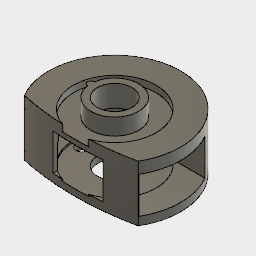
support rotacteur (Autodesk Fusion 360 design; units mm, degrees)
Autodesk Fusion 360 part; units mm, degrees
sketch "Sketch1" plane through (0, 0, 0) normal (0, 1, 0) x (1, 0, 0)
  circle A0 centre (0, 0) radius 7.25
  dimension "d1" = 14.5
  measures "d1" diameter of A0
extrude "Extrude1" add sketch "Sketch1" along normal blind 5 makes body 1
sketch "Sketch2" plane through (0, 0, 0) normal (0, 1, 0) x (1, 0, 0)
  circle A0 centre (0, 0) radius 20
  circle A1 centre (0, 0) radius 12.5
  dimension "d4" = 40
  dimension "d5" = 25
  measures "d4" diameter of A0
  measures "d5" diameter of A1
extrude "Extrude2" add sketch "Sketch2" against normal blind 15 separate body makes body 2
move_face "OffsetFaces1" offset 2 1 faces at (17.379, 0, 1.6146) on bodies 2
sketch "Sketch3" plane through (0, 5, 0) normal (0, 1, 0) x (-1, 0, 0)
  circle A0 centre (0, 0) radius 7.25
  circle A1 centre (0, 0) radius 5.25
  dimension "d9" = 10.5
  measures "d9" diameter of A1
extrude "Extrude3" cut sketch "Sketch3" against normal blind 20 contours A1 bodies 1
extrude "Extrude4" add sketch "Sketch2" against normal blind 2 contours A1 bodies 1 2
extrude "Extrude5" cut sketch "Sketch3" against normal blind 25 contours A1 bodies 1
extrude "Extrude6" add 1 faces at (10.0172, -2, 0.8818) along direction (0, -1, 0) blind 13 on bodies 1 bodies 1
cylinder "CylinderPrimitive1" add diameter 25 height 10 placed x (1, 0, 0) y (0, 0, 1) z (0, -1, 0) at (0, -15, 0) separate body makes body 3
move_body "MoveBody1" bodies 3 to x (1, 0, 0) y (0, 1, 0) z (0, 0, 1) at (0, 10, 0)
move_face "OffsetFaces2" offset -2 1 faces at (-3.3879, -15, -0.621) on bodies 3
combine "Combine1" operation cut target body 1 tool bodies 3
ref_plane "WorkPlane1" through (0, -6.5, 0) normal (0, -1, 0) x (-1, 0, 0)
sketch "Sketch5" plane through (0, -6.5, 0) normal (0, -1, 0) x (1, 0, 0)
  line L0 (-23, -8) -> (-65, -8)
  line L1 (-65, -8) -> (-65, 7)
  line L2 (-65, 7) -> (-23, 7)
  line L3 (-23, 7) -> (-23, -8)
  line L4 (-7, -22.2294) -> (8, -22.2294)
  line L5 (8, -22.2294) -> (8, -68)
  line L6 (8, -68) -> (-7, -68)
  line L7 (-7, -68) -> (-7, -22.2294)
  dimension "d21" = 15
  measures "d21" distance of L0.start L2.end
extrude "Extrude7" add sketch "Sketch5" along normal blind 6 separate body contours L0 L1 L2 L3 makes body 4
move_face "OffsetFaces3" offset 5 1 faces at (-51, -6.5, -3) on bodies 4
move_face "OffsetFaces4" offset 3 1 faces at (-51, -5.1667, 7) on bodies 4
move_face "OffsetFaces5" offset 2 1 faces at (-37, -5.1667, -8) on bodies 4
move_body "MoveBody2" bodies 4 to x (1, 0, 0) y (0, 1, 0) z (0, 0, 1) at (44, 0, 0)
extrude "Extrude8" add sketch "Sketch5" along normal blind 6 separate body contours L4 L5 L6 L7 makes body 5
extrude "Extrude9" add sketch "Sketch5" against normal blind 5 contours L4 L5 L6 L7 bodies 5
move_body "MoveBody3" bodies 5 to x (1, 0, 0) y (0, 1, 0) z (0, 0, 1) at (0, 0, 47)
combine "Combine2" operation cut target body 1 tool bodies 4 5
sketch "Sketch6" plane through (0, -15, 0) normal (0, -1, 0) x (1, 0, 0)
  circle A0 centre (0, 0) radius 10
  circle A1 centre (-10, 0) radius 1.75
  circle A2 centre (0, 0) radius 5.25
  circle A3 centre (0, 0) radius 20
extrude "Extrude10" cut sketch "Sketch6" against normal blind 5 contours A0 A1 | A0 A1 picked at (-9.4053, 0) picked at (-10.5704, -0.042) bodies 1
ref_plane "WorkPlane2" through (0, 0, 0) normal (0, -1, 0) x (1, 0, 0)
sketch "Sketch7" plane through (0, 5, 0) normal (0, 1, 0) x (1, 0, 0)
  circle A0 centre (0, 0) radius 5.25
  circle A1 centre (0, 0) radius 7.25
sketch "Sketch8" plane through (0, 5, 0) normal (0, 1, 0) x (-1, 0, 0)
  circle A0 centre (0, 0) radius 5.25
  circle A1 centre (0, 0) radius 7.25
  circle A2 centre (7.25, 0) radius 1
  point P0 (7.25, 0)
  dimension "d36" = 2
  measures "d36" diameter of A2
extrude "Extrude11" add sketch "Sketch8" against normal blind 5 contours A1 A2 picked at (7.5661, -0.2091) bodies 1
sketch "Sketch9" plane through (0, 5, 0) normal (0, 1, 0) x (-1, 0, 0)
  circle A0 centre (0, 0) radius 5.25
  arc A1 (7.181, 0.9976) -> (7.181, -0.9976) centre (0, 0) ccw
  arc A2 (7.181, -0.9976) -> (7.181, 0.9976) centre (7.25, 0) ccw
  circle A3 centre (0, 0) radius 70
  circle A4 centre (0, -70) radius 81.977
  dimension "d39" = 140
  measures "d39" diameter of A3
extrude "Extrude12" cut sketch "Sketch9" against normal blind 20 contours A3 A4 picked at (-0.3644, 31.1708) bodies 1
